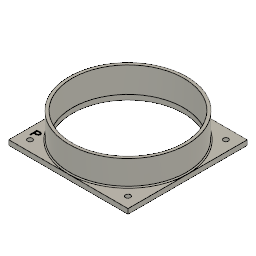
To Pipe Square (Autodesk Fusion 360 design; units mm, degrees)
Autodesk Fusion 360 part; units mm, degrees
sketch "Sketch1" plane through (0, 0, 0) normal (0, 1, 0) x (1, 0, 0)
  circle A0 centre (0, 0) radius 54.8125
  circle A1 centre (0, 0) radius 57.8125
  line L0 (59, 59) -> (-59, 59)
  line L1 (-59, 59) -> (-59, -59)
  line L2 (-59, -59) -> (59, -59)
  line L3 (59, -59) -> (59, 59)
  line L4 (59, 59) -> (-59, -59) construction
  line L5 (-59, 59) -> (59, -59) construction
  circle A2 centre (-48.3934, 48.3934) radius 2.5
  circle A3 centre (-48.3934, -48.3934) radius 2.5
  circle A4 centre (48.3934, -48.3934) radius 2.5
  circle A5 centre (48.3934, 48.3934) radius 2.5
  dimension "d7" = 109.625
  dimension "d8" = 115.625
  dimension "d9" = 118
  dimension "d10" = 118
  dimension "d11" = 5
  dimension "d12" = 15
  dimension "d15" = 0
  dimension "d16" = 0
  dimension "d18" = 360
  measures "d7" diameter of A0
  measures "d8" diameter of A1
  measures "d11" diameter of A2
ref_plane "WorkPlane1" through (0, 30, 0) normal (0, 1, 0) x (1, 0, 0)
sketch "Sketch2" plane through (0, 30, 0) normal (0, 1, 0) x (1, 0, 0)
  circle A0 centre (0, 0) radius 55.1875
  circle A1 centre (0, 0) radius 58.1875
  dimension "d20" = 110.375
  dimension "d21" = 116.375
  measures "d20" diameter of A0
  measures "d21" diameter of A1
extrude "Extrude1" add sketch "Sketch1" along normal blind 5 contours A1 | L0 L1 L2 L3
ref_plane "WorkPlane2" through (0, 5, 0) normal (0, 1, 0) x (1, 0, 0)
sketch "Sketch3" plane through (0, 5, 0) normal (0, 1, 0) x (1, 0, 0)
  line L0 (59, -59) -> (59, 59)
  circle A0 centre (0, 0) radius 57.8125
  circle A1 centre (0, 0) radius 54.8125
  line L1 (-59, 59) -> (59, -59) construction
  dimension "d25" = 109.625
  dimension "d26" = 115.625
  measures "d25" diameter of A1
  measures "d26" diameter of A0
loft "Loft1" add profiles "Sketch2", "Sketch3" section 1 section 2
loft "Loft2" cut profiles "Sketch2", "Sketch3" section 1 contours A0 section 2 contours A1
fillet "Fillet1" radius 1 1 edges at (-53.9002, 5, -20.9059)
sketch "Sketch4" plane through (0, 5, 0) normal (0, 1, 0) x (-1, 0, 0)
  line L0 (-59, 59) -> (-59, -59)
  line L1 (-59, -59) -> (59, -59)
  line L2 (59, -59) -> (59, 59)
  line L3 (59, 59) -> (-59, 59)
  circle A0 centre (48.3934, -48.3934) radius 2.5
  circle A1 centre (-48.3934, -48.3934) radius 2.5
  circle A2 centre (-48.3934, 48.3934) radius 2.5
  circle A3 centre (48.3934, 48.3934) radius 2.5
  circle A4 centre (0, 0) radius 58.8276
  line L4 (53, 44) -> (47.5361, 44) construction
  line L5 (47.5361, 44) -> (47.5361, 34) construction
  line L6 (47.5361, 34) -> (53, 34) construction
  line L7 (53, 34) -> (53, 44) construction
  text T0 "P" font "Arial" height 10 align ink ink in box 0 x 0 at (53, 44) x (-1, 0) y (0, -1) spacing 1 height is em
extrude "Extrude2" cut sketch "Sketch4" against normal blind 1 text T0
equation "ID = 110 mm"
equation "OD = ID + ( WallThickness * 2 )"
equation "WallThickness = 3 mm"
equation "Length = 30 mm"
equation "ScrewHoleDiam = 5 mm"
equation "TaperOffset = -0.75 mm"
equation "d7 = ID + ( TaperOffset / 2 )"
equation "d8 = OD + ( TaperOffset / 2 )"
equation "d11 = ScrewHoleDiam"
equation "d19 = Length"
equation "d20 = ID - ( TaperOffset / 2 )"
equation "d21 = OD - ( TaperOffset / 2 )"
equation "d25 = ID + ( TaperOffset / 2 )"
equation "d26 = OD + ( TaperOffset / 2 )"
